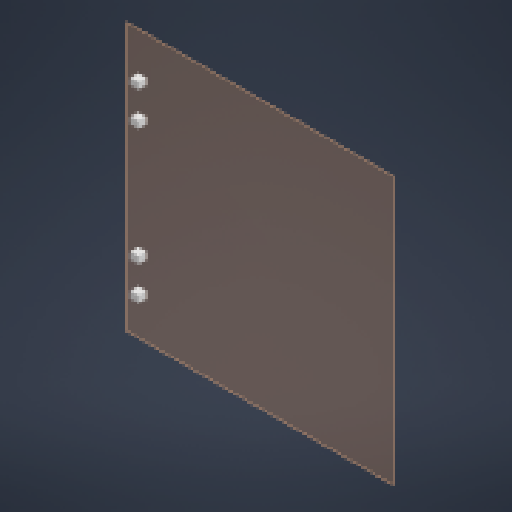
# Autodesk Inventor part: plugassholder
Saved by Autodesk Inventor 2026.2 (Build 302298010, 298A)
## iProperties
Created: 2026-09-27
Part Number: plugassholder
Material: Generic
Document SubType Name: Modeling
Designer: karol
Density: 1 g/cm^3
Appearance: Default
Author: karol
Autodesk Inventor part; units mm, degrees
ref_plane "YZ Plane" through (0, 0, 0) normal (1, 0, 0) x (0, 1, 0)
ref_plane "XZ Plane" through (0, 0, 0) normal (0, 1, 0) x (-1, 0, 0)
ref_plane "XY Plane" through (0, 0, 0) normal (0, 0, 1) x (1, 0, 0)
sketch "Sketch1" plane through (0, 0, 0) normal (0, 0, 1) x (1, 0, 0)
  line L0 (-76, -39.25) -> (-82, -39.25) projected
  line L1 (-82, -39.25) -> (-82, -20.75) projected
  line L2 (-82, -20.75) -> (-76, -20.75) projected
  line L3 (-76, -20.75) -> (-76, -39.25) projected
  line L4 (-76, 20.75) -> (-82, 20.75) projected
  line L5 (-82, 20.75) -> (-82, 39.25) projected
  line L6 (-82, 39.25) -> (-76, 39.25) projected
  line L7 (-76, 39.25) -> (-76, 20.75) projected
  circle A0 centre (-63, -65) radius 1.5 projected
  circle A1 centre (-16.6, -87) radius 1.5 projected
  circle A2 centre (49.6, -87) radius 1.5 projected
  circle A3 centre (46.6, -60) radius 1.5 projected
  circle A4 centre (87, -63) radius 1.5 projected
  circle A5 centre (46.6, -32) radius 1.5 projected
  circle A6 centre (46.6, 32) radius 1.5 projected
  circle A7 centre (87, 63) radius 1.5 projected
  circle A8 centre (46.6, 60) radius 1.5 projected
  circle A9 centre (49.6, 87) radius 1.5 projected
  circle A10 centre (-16.6, 87) radius 1.5 projected
  circle A11 centre (-16.6, 65) radius 1.5 projected
  circle A12 centre (-63, 65) radius 1.5 projected
  line L8 (-58, -60) -> (-60, -60) projected
  line L9 (-60, -60) -> (-60, -39.5) projected
  line L10 (-60, -39.5) -> (-58, -39.5) projected
  line L11 (-58, -39.5) -> (-58, -60) projected
  line L12 (49.6, 30) -> (51.6, 30) projected
  line L13 (51.6, 30) -> (51.6, 9.5) projected
  line L14 (51.6, 9.5) -> (49.6, 9.5) projected
  line L15 (49.6, 9.5) -> (49.6, 30) projected
  line L16 (-58, 39.5) -> (-60, 39.5) projected
  line L17 (-60, 39.5) -> (-60, 60) projected
  line L18 (-60, 60) -> (-58, 60) projected
  line L19 (-58, 60) -> (-58, 39.5) projected
  line L20 (-21.6, -39.5) -> (-19.6, -39.5) projected
  line L21 (-19.6, -39.5) -> (-19.6, -60) projected
  line L22 (-19.6, -60) -> (-21.6, -60) projected
  line L23 (-21.6, -60) -> (-21.6, -39.5) projected
  line L24 (51.6, -30) -> (49.6, -30) projected
  line L25 (49.6, -30) -> (49.6, -9.5) projected
  line L26 (49.6, -9.5) -> (51.6, -9.5) projected
  line L27 (51.6, -9.5) -> (51.6, -30) projected
  line L28 (-21.6, 60) -> (-19.6, 60) projected
  line L29 (-19.6, 60) -> (-19.6, 39.5) projected
  line L30 (-19.6, 39.5) -> (-21.6, 39.5) projected
  line L31 (-21.6, 39.5) -> (-21.6, 60) projected
  line L32 (90, -35) -> (90, 35) projected
  line L33 (90, 35) -> (49.6, 35) projected
  line L34 (49.6, 35) -> (49.6, 60) projected
  line L35 (49.6, 60) -> (90, 60) projected
  line L36 (90, 60) -> (90, 90) projected
  line L37 (90, 90) -> (-19.6, 90) projected
  line L38 (-19.6, 90) -> (-19.6, 65) projected
  line L39 (-19.6, 65) -> (-60, 65) projected
  line L40 (-60, 65) -> (-60, 90) projected
  line L41 (-60, 90) -> (-90, 90) projected
  line L42 (-90, 90) -> (-90, -90) projected
  line L43 (-90, -90) -> (-60, -90) projected
  line L44 (-60, -90) -> (-60, -65) projected
  line L45 (-60, -65) -> (-19.6, -65) projected
  line L46 (-19.6, -65) -> (-19.6, -90) projected
  line L47 (-19.6, -90) -> (90, -90) projected
  line L48 (90, -90) -> (90, -60) projected
  line L49 (90, -60) -> (49.6, -60) projected
  line L50 (49.6, -60) -> (49.6, -35) projected
  line L51 (49.6, -35) -> (90, -35) projected
  line L52 (86, -32) -> (73.8, -32) projected
  line L53 (73.8, -32) -> (73.8, -7.5) projected
  line L54 (73.8, -7.5) -> (86, -7.5) projected
  line L55 (86, -7.5) -> (86, -32) projected
  line L56 (65.8, -32) -> (53.6, -32) projected
  line L57 (53.6, -32) -> (53.6, -7.5) projected
  line L58 (53.6, -7.5) -> (65.8, -7.5) projected
  line L59 (65.8, -7.5) -> (65.8, -32) projected
  line L60 (86, -86) -> (70.6, -86) projected
  line L61 (70.6, -86) -> (70.6, -69.8) projected
  line L62 (70.6, -69.8) -> (86, -69.8) projected
  line L63 (86, -69.8) -> (86, -86) projected
  line L64 (86, 86) -> (86, 69.8) projected
  line L65 (86, 69.8) -> (70.6, 69.8) projected
  line L66 (70.6, 69.8) -> (70.6, 86) projected
  line L67 (70.6, 86) -> (86, 86) projected
  line L68 (73.8, 32) -> (86, 32) projected
  line L69 (86, 32) -> (86, 7.5) projected
  line L70 (86, 7.5) -> (73.8, 7.5) projected
  line L71 (73.8, 7.5) -> (73.8, 32) projected
  line L72 (65.8, 32) -> (65.8, 7.5) projected
  line L73 (65.8, 7.5) -> (53.6, 7.5) projected
  line L74 (53.6, 7.5) -> (53.6, 32) projected
  line L75 (53.6, 32) -> (65.8, 32) projected
  line L76 (-69.6, -87) -> (-85, -87) projected
  line L77 (-85, -87) -> (-85, -70.8) projected
  line L78 (-85, -70.8) -> (-69.6, -70.8) projected
  line L79 (-69.6, -70.8) -> (-69.6, -87) projected
  line L80 (-56, -62) -> (-56, -37.5) projected
  line L81 (-56, -37.5) -> (-43.8, -37.5) projected
  line L82 (-43.8, -37.5) -> (-43.8, -62) projected
  line L83 (-43.8, -62) -> (-56, -62) projected
  line L84 (-56, 62) -> (-43.8, 62) projected
  line L85 (-43.8, 62) -> (-43.8, 37.5) projected
  line L86 (-43.8, 37.5) -> (-56, 37.5) projected
  line L87 (-56, 37.5) -> (-56, 62) projected
  line L88 (-23.6, 62) -> (-23.6, 37.5) projected
  line L89 (-23.6, 37.5) -> (-35.8, 37.5) projected
  line L90 (-35.8, 37.5) -> (-35.8, 62) projected
  line L91 (-35.8, 62) -> (-23.6, 62) projected
  line L92 (-23.6, -62) -> (-35.8, -62) projected
  line L93 (-35.8, -62) -> (-35.8, -37.5) projected
  line L94 (-35.8, -37.5) -> (-23.6, -37.5) projected
  line L95 (-23.6, -37.5) -> (-23.6, -62) projected
  line L96 (-85, 87) -> (-69.6, 87) projected
  line L97 (-69.6, 87) -> (-69.6, 70.8) projected
  line L98 (-69.6, 70.8) -> (-85, 70.8) projected
  line L99 (-85, 70.8) -> (-85, 87) projected
  line L100 (-90, 70.8) -> (-84, 70.8)
  line L101 (-84, 70.8) -> (-84, -70.8)
  line L102 (-84, -70.8) -> (-90, -70.8)
  line L103 (-90, -70.8) -> (-90, 70.8)
  line L104 (-84, -70.8) -> (-90, -70.8)
  line L105 (-90, -70.8) -> (-90, -65.8)
  line L106 (-90, -65.8) -> (-84, -65.8)
  line L107 (-84, -65.8) -> (-84, -70.8)
  line L108 (-84, -65.8) -> (-90, -65.8)
  line L109 (-90, -65.8) -> (-90, -45.8)
  line L110 (-90, -45.8) -> (-84, -45.8)
  line L111 (-84, -45.8) -> (-84, -65.8)
  line L112 (-84, -45.8) -> (-90, -45.8)
  line L113 (-90, -45.8) -> (-90, -40.8)
  line L114 (-90, -40.8) -> (-84, -40.8)
  line L115 (-84, -40.8) -> (-84, -45.8)
  line L116 (-90, 0) -> (-84, 0)
  line L117 (-84, 70.8) -> (-90, 70.8)
  line L118 (-84, 70.8) -> (-90, 70.8)
  line L119 (-90, 70.8) -> (-90, 65.8)
  line L120 (-90, 65.8) -> (-84, 65.8)
  line L121 (-84, 65.8) -> (-84, 70.8)
  line L122 (-84, 65.8) -> (-90, 65.8)
  line L123 (-90, 65.8) -> (-90, 45.8)
  line L124 (-90, 45.8) -> (-84, 45.8)
  line L125 (-84, 45.8) -> (-84, 65.8)
  line L126 (-84, 45.8) -> (-90, 45.8)
  line L127 (-90, 45.8) -> (-90, 40.8)
  line L128 (-90, 40.8) -> (-84, 40.8)
  line L129 (-84, 40.8) -> (-84, 45.8)
  point P0 (0, 0)
  point P1 (-87, -70.8)
  point P2 (-87, 70.8)
  dimension "d0" = 6
  dimension "d1" = 6
  dimension "d2" = 5
  dimension "d3" = 20
  dimension "d4" = 6
  dimension "d5" = 5
  dimension "d6" = 0
  constraints: 60 end point, 13 symmetric about line, 8 parallel, 4 horizontal, 4 perpendicular, 4 point on line, 3 midpoint
  measures "d0" distance of L101.end L102.end
  measures "d1" distance of L105.end L106.end
  measures "d2" distance of L104.end L105.end
  measures "d3" distance of L108.end L109.end
  measures "d4" distance of L113.end L114.end
  measures "d5" distance of L112.end L113.end
  measures "d6" distance from line of point (-87, -70.8) L104
extrude "Extrusion1" add sketch "Sketch1" along normal blind 5.8 contours L42 L106 L101 L78 L102 | L100 L98 L101 L120 L42 | L42 L114 L101 L110 | L124 L101 L128 L42
ref_plane "Work Plane1" through (0, 0, 0) normal (0, 0, 1) x (1, 0, 0)
sketch "Sketch2" plane through (0, 0, 0) normal (0, 0, 1) x (1, 0, 0)
  line L0 (-84, 40.8) -> (-84, 45.8) projected
  line L1 (-84, 45.8) -> (-90, 45.8) projected
  line L2 (-90, 45.8) -> (-90, 40.8) projected
  line L3 (-90, 40.8) -> (-84, 40.8) projected
  line L4 (-90, -40.8) -> (-90, -45.8) projected
  line L5 (-90, -45.8) -> (-84, -45.8) projected
  line L6 (-84, -45.8) -> (-84, -40.8) projected
  line L7 (-84, -40.8) -> (-90, -40.8) projected
  line L8 (-84, 65.8) -> (-84, 70.8) projected
  line L9 (-84, 70.8) -> (-90, 70.8) projected
  line L10 (-90, 70.8) -> (-90, 65.8) projected
  line L11 (-90, 65.8) -> (-84, 65.8) projected
  line L12 (-90, -65.8) -> (-90, -70.8) projected
  line L13 (-90, -70.8) -> (-84, -70.8) projected
  line L14 (-84, -70.8) -> (-84, -65.8) projected
  line L15 (-84, -65.8) -> (-90, -65.8) projected
  line L16 (-84, -65.8) -> (-90, -65.8)
  line L17 (-90, -65.8) -> (-90, -45.8)
  line L18 (-90, -45.8) -> (-84, -45.8)
  line L19 (-84, -45.8) -> (-84, -65.8)
  line L20 (-90, -40.8) -> (-84, -40.8)
  line L21 (-84, -40.8) -> (-84, 40.8)
  line L22 (-84, 40.8) -> (-90, 40.8)
  line L23 (-90, 40.8) -> (-90, -40.8)
  line L24 (-90, 65.8) -> (-84, 65.8)
  line L25 (-84, 65.8) -> (-84, 45.8)
  line L26 (-84, 45.8) -> (-90, 45.8)
  line L27 (-90, 45.8) -> (-90, 65.8)
  point P0 (0, 0)
  constraints: 24 end point, 6 parallel, 3 horizontal, 3 perpendicular
extrude "Extrusion2" add sketch "Sketch2" along normal blind 1 contours L21 L7 L23 L3 | L1 L27 L11 L25 | L19 L15 L17 L5
fillet "Fillet1" radius 2.5 8 edges at (-84, -68.3, 5.8) (-90, -68.3, 5.8) (-90, -43.3, 5.8) (-84, -43.3, 5.8) (-84, 43.3, 5.8) (-90, 43.3, 5.8) (-90, 68.3, 5.8) (-84, 68.3, 5.8)
sketch "Sketch3" plane through (-90, -70.8, 0) normal (0, -1, 0) x (1, 0, 0)
  circle A0 centre (3, 3.6) radius 1.2
  line L0 (6, 0) -> (6, 3.3) projected
  line L1 (0, 0) -> (6, 0) projected
  point P0 (90, 0)
  dimension "d12" = 2.4
  dimension "d13" = 3
  dimension "d14" = 3.6
  constraints: 1 centre point
  measures "d12" diameter of A0
  measures "d13" distance from line of L0 A0.centre
  measures "d14" distance from line of L1 A0.centre
extrude "Extrusion3" cut sketch "Sketch3" against normal blind 5
sketch "Sketch4" plane through (-90, -45.8, 1) normal (0, -1, 0) x (1, 0, 0)
  circle A0 centre (3, 2.6) radius 1.2 projected
  point P0 (90, -1)
extrude "Extrusion4" cut sketch "Sketch4" against normal blind 5
sketch "Sketch5" plane through (-90, 40.8, 1) normal (0, -1, 0) x (1, 0, 0)
  circle A0 centre (3, 2.6) radius 1.2 projected
  point P0 (90, -1)
extrude "Extrusion5" cut sketch "Sketch5" against normal blind 5
sketch "Sketch6" plane through (-90, 65.8, 1) normal (0, -1, 0) x (1, 0, 0)
  circle A0 centre (3, 2.6) radius 1.2 projected
  point P0 (90, -1)
extrude "Extrusion6" cut sketch "Sketch6" against normal blind 5
body "Solid1"
